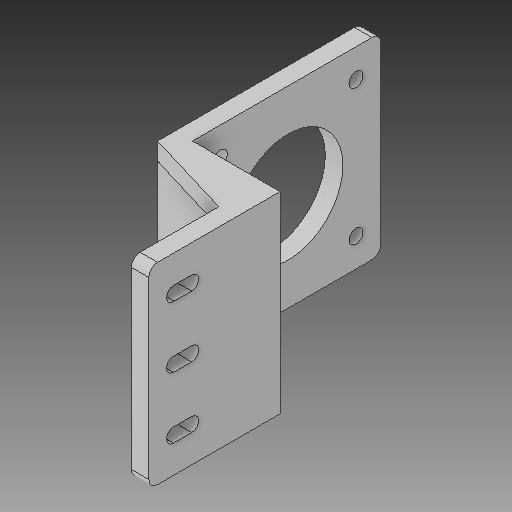
# Autodesk Inventor part: MotorMountZaxis
Saved by Autodesk Inventor 2018 (Build 220112000, 112)
## iProperties
Created: 2017-10-07
Part Number: MotorMountZaxis
Material: Generic
Document SubType Name: Modeling
Designer: Jurjen
Density: 1 g/cm^3
Appearance: Default
Author: Jurjen
Autodesk Inventor part; units mm, degrees
ref_plane "YZ Plane" through (0, 0, 0) normal (1, 0, 0) x (0, 1, 0)
ref_plane "XZ Plane" through (0, 0, 0) normal (0, 1, 0) x (-1, 0, 0)
ref_plane "XY Plane" through (0, 0, 0) normal (0, 0, 1) x (1, 0, 0)
sketch "Sketch1" plane through (0, 0, 0) normal (0, 1, 0) x (-1, 0, 0)
  line L0 (-6, 20) -> (-6, 0)
  line L1 (-6, 0) -> (14, -6)
  line L2 (14, -6) -> (14, -53)
  line L3 (14, -53) -> (10, -53)
  line L4 (10, -53) -> (10, -10)
  line L5 (-10, -10) -> (-10, 20)
  line L6 (-10, 20) -> (-6, 20)
  line L7 (10, -10) -> (-10, -10)
  point P0 (0, 0)
  point P1 (0, -10)
  dimension "d0" = 20
  dimension "d1" = 43
  dimension "d2" = 4
  dimension "d3" = 4
  dimension "d4" = 30
  dimension "d5" = 20
  dimension "d6" = 4
  constraints: 16 end point, 2 horizontal, 2 parallel, 2 perpendicular, 1 horizontal alignment, 1 midpoint, 1 vertical, 1 vertical alignment
  measures "d0" distance of L4.end L5.start
  measures "d1" distance of L3.end L4.end
  measures "d2" distance of L2.end L3.end
  measures "d3" distance of L5.end L0.start
  measures "d4" distance of L5.start L5.end
  measures "d5" distance of L0.start L0.end
  measures "d6" distance from line of L1.end L7
extrude "Extrusion1" add sketch "Sketch1" along normal mid plane 44
sketch "Sketch2" plane through (-14, -22, -6) normal (-1, 0, 0) x (0, 0, 1)
  line L0 (0, 44) -> (0, 0) projected
  line L1 (-47, 44) -> (0, 44) projected
  line L2 (-47, 44) -> (-47, 0) projected
  line L3 (0, 0) -> (-47, 0) projected
  circle A0 centre (-25.85, 22) radius 12.5
  circle A1 centre (-41.35, 37.5) radius 1.6
  circle A2 centre (-41.35, 6.5) radius 1.6
  circle A3 centre (-10.35, 37.5) radius 1.6
  circle A4 centre (-10.35, 6.5) radius 1.6
  point P0 (6, 22)
  point P1 (-47, 22)
  dimension "d9" = 3.2
  dimension "d10" = 25
  dimension "d11" = 21.15
  dimension "d12" = 31
  dimension "d13" = 31
  dimension "d14" = 15.5
  dimension "d15" = 15.5
  constraints: 5 centre point, 3 equal radius, 3 horizontal alignment, 2 vertical alignment, 1 midpoint
  measures "d9" diameter of A1
  measures "d10" diameter of A0
  measures "d11" distance from line of L2 A0.centre
  measures "d12" distance of A1.centre A2.centre
  measures "d13" distance of A1.centre A3.centre
  measures "d14" horizontal distance of A0.centre A1.centre
  measures "d15" horizontal distance of A1.centre A0.centre
extrude "Extrusion2" cut sketch "Sketch2" against normal up to next contours A0 | A1 | A2 | A3 | A4
sketch "Sketch3" plane through (6, -22, 20) normal (-1, 0, 0) x (0, 0, 1)
  arc A0 (-5.7957, 34.4085) -> (-5.6306, 37.6) centre (-5.6306, 36) ccw
  arc A1 (-9.6306, 37.6) -> (-9.7957, 34.4085) centre (-9.7957, 36.0085) ccw
  arc A2 (-5.6306, 20.4) -> (-5.6306, 23.6) centre (-5.6306, 22) ccw
  arc A3 (-9.7957, 23.6) -> (-9.7957, 20.4) centre (-9.7957, 22) ccw
  arc A4 (-5.6306, 6.4) -> (-5.6306, 9.6) centre (-5.6306, 8) ccw
  arc A5 (-9.7957, 9.6) -> (-9.7957, 6.4) centre (-9.7957, 8) ccw
  line L0 (-9.6306, 37.6) -> (-5.6306, 37.6)
  line L1 (-9.7957, 34.4085) -> (-5.7957, 34.4085)
  line L2 (-9.7957, 23.6) -> (-5.6306, 23.6)
  line L3 (-9.7957, 20.4) -> (-5.6306, 20.4)
  line L4 (-9.7957, 9.6) -> (-5.6306, 9.6)
  line L5 (-9.7957, 6.4) -> (-5.6306, 6.4)
  line L6 (-20, 44) -> (0, 44) projected
  line L7 (0, 0) -> (-20, 0) projected
  line L8 (-5.6306, 36) -> (-5.6306, 8) construction
  point P0 (-20, 22)
  dimension "d18" = 3.2
  dimension "d19" = 4
  dimension "d20" = 8
  dimension "d21" = 8
  constraints: 14 end point, 12 point on circle, 6 centre point, 5 equal radius, 5 parallel, 4 vertical alignment, 2 tangent, 1 coincident, 1 horizontal, 1 midpoint, 1 vertical
  measures "d18" diameter of A0
  measures "d19" distance of L0.start L0.end
  measures "d20" distance from line of L6 L8.start
  measures "d21" distance from line of L7 L8.end
extrude "Extrusion3" cut sketch "Sketch3" against normal up to next
sketch "Sketch4" plane through (-14, -22, -6) normal (-1, 0, 0) x (0, 0, 1)
  line L0 (0, 44) -> (0, 0) projected
  line L1 (0, 40) -> (8.5563, 40)
  line L2 (8.5563, 40) -> (8.5563, 4)
  line L3 (8.5563, 4) -> (0, 4)
  line L4 (0, 4) -> (0, 40)
  point P0 (6, 22)
  dimension "d26" = 4
  dimension "d27" = 4
  constraints: 8 end point, 2 parallel, 1 horizontal, 1 perpendicular, 1 point on line
  measures "d26" distance from line of L0.start L1
  measures "d27" distance from line of L0.end L3
extrude "Extrusion4" cut sketch "Sketch4" against normal up to surface (20 mm away)
fillet "Fillet1" radius 2 4 edges at (-12, 22, -53) (-12, -22, -53) (8, -22, 20) (8, 22, 20)
equation "\"d14\" = 0.5 * d13"
equation "\"d15\" = 0.5 * d12"
body "Solid1"
